Autodesk Fusion 360 part; units mm, degrees
(part 2 of 5)
  spline S0 degree 3 poles (45.4352, 19.4331, 2.5409) (44.7866, 20.9539, 2.7513) (44.0616, 22.4421, 2.9616) (43.2623, 23.8896, 3.172) (39.2446, 31.1652, 4.2293) (33.358, 37.3986, 5.2866) (26.324, 41.8256, 6.3439) (19.2902, 46.2525, 7.4011) (11.1241, 48.8637, 8.4584) (2.8268, 49.3391, 9.5157) (-5.4704, 49.8145, 10.5729) (-13.8811, 48.1531, 11.6302) (-21.3743, 44.5587, 12.6874) (-28.8674, 40.9643, 13.7447) (-35.4271, 35.4447, 14.8019) (-40.2493, 28.6763, 15.8591) (-45.0715, 21.908, 16.9163) (-48.146, 13.9055, 17.9735) (-49.096, 5.6496, 19.0307) (-50.046, -2.606, 20.0879) (-48.8696, -11.0975, 21.1451) (-45.711, -18.784, 22.2022) (-42.5525, -26.4703, 23.2594) (-37.4186, -33.3353, 24.3165) (-30.9385, -38.5376, 25.3737) (-24.4586, -43.7398, 26.4308) (-16.6463, -47.2683, 27.4879) (-8.4592, -48.6906, 28.545) (-0.2722, -50.113, 29.6021) (8.2721, -49.4263, 30.6592) (16.1268, -46.7147, 31.7163) (23.9813, -44.0032, 32.7734) (31.1295, -39.2726, 33.8305) (36.6953, -33.1027, 34.8876) (42.261, -26.933, 35.9446) (46.2326, -19.3372, 37.0017) (48.1234, -11.246, 38.0587) (50.0142, -3.155, 39.1157) (49.8203, 5.4141, 40.1728) (47.5655, 13.4113, 41.2298) (45.3107, 21.4083, 42.2868) (40.9999, 28.8164, 43.3438) (35.1612, 34.7279, 44.4008) (29.3227, 40.6393, 45.4577) (21.9688, 45.0415, 46.5147) (14.0006, 47.3954, 47.5717) (6.0326, 49.7491, 48.6286) (-2.5328, 50.0495, 49.6856) (-10.6461, 48.2597, 50.7425) (-18.7593, 46.4699, 51.7995) (-26.4031, 42.5939, 52.8564) (-32.6413, 37.1064, 53.9133) (-38.8792, 31.6191, 54.9702) (-43.6983, 24.5321, 56.0271) (-46.508, 16.7136, 57.084) (-49.3176, 8.8953, 58.1409) (-50.1121, 0.3622, 59.1978) (-48.7941, -7.8404, 60.2546) (-47.4761, -16.0429, 61.3115) (-44.0485, -23.8973, 62.3684) (-38.9312, -30.4418, 63.4252) (-33.8139, -36.986, 64.482) (-27.0179, -42.2064, 65.5389) (-19.3756, -45.4634, 66.5957) (-11.7334, -48.7204, 67.6525) (-3.2612, -50.0071, 68.7093) (5.0034, -49.1661, 69.7661) (13.2677, -48.3251, 70.8229) (21.3069, -45.3581, 71.8796) (28.1362, -40.6287, 72.9364) (34.9654, -35.8993, 73.9932) (40.5702, -29.4176, 75.0499) (44.2643, -21.9774, 76.1067) (47.9584, -14.5373, 77.1634) (49.7339, -6.1545, 78.2202) (49.3735, 2.1444, 79.2769) (49.013, 10.4431, 80.3336) (46.5175, 18.6401, 81.3903) (42.1925, 25.7318, 82.447) (37.8676, 32.8234, 83.5037) (31.7225, 38.7945, 84.5604) (24.5097, 42.914, 85.617) (17.2971, 47.0334, 86.6737) (9.0322, 49.2925, 87.7304) (0.7269, 49.4147, 88.787) (-7.5781, 49.5368, 89.8437) (-15.9057, 47.5219, 90.9003) (-23.2363, 43.6166, 91.9569) (-30.5667, 39.7114, 93.0135) (-36.8845, 33.9243, 94.0701) (-41.4161, 26.9637, 95.1268) (-45.9477, 20.0033, 96.1833) (-48.6835, 11.8843, 97.2399) (-49.2886, 3.6009, 98.2965) (-49.8938, -4.6824, 99.3531) (-48.3671, -13.1126, 100.4096) (-44.8954, -20.6576, 101.4662) (-41.4239, -28.2024, 102.5227) (-36.0148, -34.846, 103.5793) (-29.3305, -39.7751, 104.6358) (-22.6463, -44.7041, 105.6923) (-14.7012, -47.9081, 106.7488) (-6.4676, -48.995, 107.8054) (1.7658, -50.0818, 108.8619) (10.27, -49.0493, 109.9183) (18.0041, -46.0238, 110.9748) (25.738, -42.9983, 112.0313) (32.6854, -37.9864, 113.0878) (37.9957, -31.6016, 114.1442) (43.306, -25.2168, 115.2007) (46.9681, -17.4728, 116.2571) (48.5337, -9.3173, 117.3136) (50.0994, -1.1619, 118.37) (49.5653, 7.3875, 119.4264) (46.997, 15.2846, 120.4828) (44.4287, 23.1815, 121.5392) (39.8317, 30.4094, 122.5956) (33.7686, 36.0835, 123.652) (27.7056, 41.7575, 124.7084) (20.1894, 45.8659, 125.7648) (12.14, 47.9057, 126.8211) (4.0907, 49.9455, 127.8775) (-4.4747, 49.9126, 128.9338) (-12.508, 47.8109, 129.9902) (-20.5412, 45.7093, 131.0465) (-28.0252, 41.5436, 132.1029) (-34.0443, 35.8235, 133.1592) (-40.0632, 30.1035, 134.2155) (-44.6044, 22.8414, 135.2718) (-47.1122, 14.9259, 136.3281) (-49.6199, 7.0105, 137.3844) (-50.0889, -1.5416, 138.4407) (-48.462, -9.6838, 139.4969) (-46.835, -17.8258, 140.5532) (-43.1155, -25.5407, 141.6095) (-37.7587, -31.8844, 142.6657) (-32.402, -38.2281, 143.7219) (-25.4193, -43.1872, 144.7782) (-17.665, -46.155, 145.8344) (-9.911, -49.1227, 146.8906) (-1.4018, -50.093, 147.9468) (6.8213, -48.947, 149.0031) (15.0443, -47.801, 150.0592) (22.9638, -44.5413, 151.1154) (29.6109, -39.5668, 152.1716) (36.2579, -34.5923, 153.2278) (41.6184, -27.9136, 154.284) (45.0367, -20.3478, 155.3401) (48.4549, -12.782, 156.3963) (49.9237, -4.3452, 157.4524) (49.2634, 3.9305, 158.5085) (48.6032, 12.2061, 159.5647) (45.8153, 20.3031, 160.6208) (41.2409, 27.231, 161.6769) (36.6665, 34.1588, 162.733) (30.3154, 39.9028, 163.7891) (22.9644, 43.7604, 164.8452) (15.6136, 47.6179, 165.9013) (7.2785, 49.581, 166.9574) (-1.0213, 49.4094, 168.0134) (-9.3208, 49.2379, 169.0695) (-17.5675, 46.9322, 170.1255) (-24.7525, 42.7744, 171.1816) (-31.9374, 38.6166, 172.2376) (-38.0455, 32.6157, 173.2936) (-42.3297, 25.5055, 174.3497) (-46.6139, 18.3954, 175.4057) (-49.0651, 10.1912, 176.4617) (-49.3836, 1.8964, 177.5177) (-49.7021, -6.3984, 178.5737) (-47.8874, -14.7662, 179.6297) (-44.1613, -22.1837, 180.6857) (-40.4353, -29.6011, 181.7416) (-34.8059, -36.0525, 182.7976) (-27.9617, -40.749, 183.8535) (-21.1176, -45.4454, 184.9095) (-13.0731, -48.3769, 185.9654) (-4.8121, -49.1852, 187.0214) (3.4487, -49.9934, 188.0773) (11.9086, -48.6766, 189.1332) (19.5331, -45.396, 190.1891) (27.1574, -42.1154, 191.245) (33.9301, -36.8779, 192.3009) (39.023, -30.324, 193.3568) (44.1158, -23.7702, 194.4127) (47.5181, -15.9139, 195.4685) (48.814, -7.7157, 196.5244) (50.1098, 0.4823, 197.5803) (49.2964, 9.0047, 198.6361) (46.4733, 16.8097, 199.692) (43.6503, 24.6144, 200.7478) (38.8237, 31.685, 201.8036) (32.5835, 37.1571, 202.8595) (26.3435, 42.6291, 203.9153) (18.7032, 46.4909, 204.9711) (10.5968, 48.2705, 206.0269) (2.4906, 50.0501, 207.0827) (-6.0645, 49.7437, 208.1385) (-14.0227, 47.3888, 209.1942) (-21.9807, 45.034, 210.25) (-29.3248, 40.6358, 211.3058) (-35.1573, 34.7318, 212.3615) (-40.9897, 28.828, 213.4173) (-45.2981, 21.431, 214.473) (-47.5559, 13.4451, 215.5287) (-49.8137, 5.4594, 216.5845) (-50.0161, -3.0982, 217.6402) (-48.1384, -11.1818, 218.6959) (-46.2608, -19.2651, 219.7516) (-42.3071, -26.8572, 220.8073) (-36.7607, -33.0301, 221.863) (-31.2145, -39.2028, 222.9187) (-24.0873, -43.9432, 223.9744) (-16.2504, -46.6719, 225.03) (-8.4136, -49.4005, 226.0857) (0.1163, -50.1117, 227.1413) (8.2968, -48.7186, 228.197) (16.477, -47.3255, 229.2526) (24.2905, -43.8311, 230.3083) (30.7823, -38.6625, 231.3639) (37.2739, -33.4939, 232.4195) (42.4301, -26.6622, 233.4751) (45.6207, -19.0023, 234.5307) (48.8112, -11.3425, 235.5863) (50.0295, -2.8707, 236.6419) (49.1265, 5.3778, 237.6975) (48.2236, 13.6261, 238.7531) (45.2015, 21.6335, 239.8086) (40.4296, 28.4216, 240.8642) (35.6577, 35.2095, 241.9197) (29.1462, 40.7637, 242.9753) (21.6908, 44.4055, 244.0308) (14.2354, 48.0472, 245.0864) (5.852, 49.7688, 246.1419) (-2.4351, 49.36, 247.1974) (-10.7221, 48.9511, 248.2529) (-18.8952, 46.4128, 249.3084) (-25.9558, 42.0551, 250.3639) (-33.0162, 37.6976, 251.4194) (-38.9492, 31.5299, 252.4749) (-43.0298, 24.3059, 253.5304) (-47.1103, 17.082, 254.5858) (-49.3298, 8.817, 255.6413) (-49.4173, 0.5207, 256.6968) (-49.5047, -7.7753, 257.7522) (-47.4599, -16.0851, 258.8076) (-43.5326, -23.3933, 259.8631) (-39.6055, -30.7013, 260.9185) (-33.8043, -36.9923, 261.9739) (-26.8379, -41.4977, 263.0293) (-19.8716, -46.0031, 264.0847) (-11.7549, -48.7133, 265.1401) (-3.4792, -49.2974, 266.1955) (4.7962, -49.8814, 267.2509) (13.213, -48.3381, 268.3063) (20.7429, -44.8561, 269.3617) (28.2727, -41.3741, 270.417) (34.8997, -35.9607, 271.4724) (39.8143, -29.2773, 272.5277) (44.7288, -22.594, 273.5831) (47.9207, -14.6548, 274.6384) (49, -6.4296, 275.6937) (50.0792, 1.7954, 276.749) (49.0437, 10.2891, 277.8044) (46.0199, 18.0139, 278.8597) (42.9962, 25.7386, 279.915) (37.9907, 32.6781, 280.9703) (31.6148, 37.9848, 282.0256) (25.2389, 43.2914, 283.0808) (17.5063, 46.954, 284.1361) (9.3612, 48.5253, 285.1914) (1.2163, 50.0966, 286.2466) (-7.3237, 49.5733, 287.3019) (-15.2158, 47.0193, 288.3571) (-23.1077, 44.4654, 289.4124) (-30.3351, 39.8864, 290.4676) (-36.0152, 33.8414, 291.5228) (-41.6952, 27.7965, 292.578) (-45.816, 20.2986, 293.6333) (-47.8743, 12.2633, 294.6885) (-49.9325, 4.2281, 295.7437) (-49.924, -4.3274, 296.7988) (-47.8498, -12.3584, 297.854) (-45.7756, -20.3893, 298.9092) (-41.6402, -27.8788, 299.9644) (-35.9486, -33.9122, 301.0195) (-30.257, -39.9455, 302.0747) (-23.0213, -44.5101, 303.1298) (-15.1251, -47.0486, 304.185) (-7.229, -49.587, 305.2401) (1.311, -50.094, 306.2953) (9.452, -48.5077, 307.3504) (17.5928, -46.9214, 308.4055) (25.3175, -43.2452, 309.4606) (31.6828, -37.9281, 310.5157) (38.048, -32.611, 311.5708) (43.0403, -25.6642, 312.6259) (46.0504, -17.9359, 313.681) (49.0604, -10.2078, 314.736) (50.0817, -1.7145, 315.7911) (48.9898, 6.5069, 316.8462) (47.8978, 14.7282, 317.9012) (44.6949, 22.6602, 318.9563) (39.7721, 29.3346, 320.0113) (34.8494, 36.0088, 321.0664) (28.2172, 41.4114, 322.1214) (20.6853, 44.8827, 323.1764) (13.1536, 48.3539, 324.2314) (4.7381, 49.8865, 325.2864) (-3.5338, 49.2935, 326.3414) (-11.8056, 48.7005, 327.3964) (-19.9163, 45.9832, 328.4514) (-26.8757, 41.4733, 329.5064) (-33.8351, 36.9634, 330.5614) (-39.6286, 30.6706, 331.6163) (-43.5489, 23.3629, 332.6713) (-47.4692, 16.0554, 333.7263) (-49.5082, 7.7486, 334.7812) (-49.417, -0.5436, 335.8362) (-49.3258, -8.8356, 336.8911) (-47.1047, -17.0954, 337.946) (-43.0247, -24.3148, 339.0009) (-38.9448, -31.5341, 340.0558) (-33.0148, -37.6978, 341.1108) (-25.9585, -42.0534, 342.1657) (-18.9024, -46.409, 343.2206) (-10.7348, -48.9475, 344.2754) (-2.4529, -49.3591, 345.3303) (5.829, -49.7706, 346.3852) (14.2078, -48.0545, 347.4401) (21.6609, -44.4201, 348.4949) (29.1139, -40.7857, 349.5498) (35.6255, -35.2408, 350.6046) (40.401, -28.4622, 351.6595) (45.1764, -21.6836, 352.7143) (48.2057, -13.6857, 353.7692) (49.1192, -5.4444, 354.824) (50.0326, 2.7967, 355.8788) (48.8284, 11.2637, 356.9336) (45.6535, 18.9234, 357.9884) (42.4786, 26.5829, 359.0432) (37.3398, 33.4189, 360.098) (30.8642, 38.5971, 361.1528) (24.3887, 43.7753, 362.2076) (16.5901, 47.2848, 363.2623) (8.42, 48.6974, 364.3171) (0.2501, 50.11, 365.3719) (-8.274, 49.4229, 366.4266) (-16.1121, 46.7198, 367.4814) (-23.9501, 44.0167, 368.5361) (-31.0856, 39.3035, 369.5908) (-36.6479, 33.1552, 370.6456) (-42.2101, 27.0071, 371.7003) (-46.1875, 19.4369, 372.755) (-48.0946, 11.3684, 373.8097) (-50.0018, 3.3001, 374.8644) (-49.8349, -5.2495, 375.9191) (-47.6142, -13.2373, 376.9738) (-45.3936, -21.2249, 378.0285) (-41.1239, -28.6337, 379.0831) (-35.3263, -34.56, 380.1378) (-29.5287, -40.4861, 381.1925) (-22.2154, -44.9171, 382.2471) (-14.2786, -47.3123, 383.3018) (-6.3419, -49.7076, 384.3564) (2.2015, -50.0621, 385.4111) (10.3093, -48.3327, 386.4657) (18.417, -46.6034, 387.5203) (26.072, -42.7938, 388.5749) (32.3406, -37.3688, 389.6296) (38.609, -31.9438, 390.6842) (43.4777, -24.9149, 391.7388) (46.3527, -17.1395, 392.7933) (49.2277, -9.3642, 393.8479) (50.1031, -0.8589, 394.9025) (48.872, 7.339, 395.9571) (47.641, 15.5367, 397.0117) (44.3062, 23.4097, 398.0662) (39.2745, 29.9975, 399.1208) (34.2428, 36.5852, 400.1753) (27.5249, 41.874, 401.2299) (19.9401, 45.2187, 402.2844) (12.3555, 48.5633, 403.3389) (3.9201, 49.9568, 404.3935) (-4.3373, 49.2293, 405.448) (-12.5945, 48.5018, 406.5025) (-20.6562, 45.6549, 407.557) (-27.5391, 41.0358, 408.6115) (-34.4219, 36.4167, 409.666) (-40.1114, 30.0353, 410.7205) (-43.9137, 22.6698, 411.775) (-47.716, 15.3044, 412.8294) (-49.6231, 6.9705, 413.8839) (-49.4025, -1.3154, 414.9384) (-49.1819, -9.6012, 415.9928) (-46.834, -17.8217, 417.0473) (-42.6454, -24.9742, 418.1017) (-38.4567, -32.1266, 419.1561) (-32.4362, -38.196, 420.2106) (-25.3179, -42.4422, 421.265) (-18.1997, -46.6884, 422.3194) (-9.9988, -49.1025, 423.3738) (-1.7153, -49.3902, 424.4282) (6.568, -49.6779, 425.4826) (14.9165, -47.8386, 426.537) (22.312, -44.0966, 427.5914) (29.7074, -40.3547, 428.6458) (36.1343, -34.7181, 429.7002) (40.809, -27.874, 430.7546) (45.4837, -21.0301, 431.8089) (48.3963, -12.9933, 432.8633) (49.1918, -4.7435, 433.9176) (49.9873, 3.5061, 434.972) (48.6641, 11.9513, 436.0263) (45.3834, 19.5622, 437.0806) (42.1028, 27.173, 438.135) (36.8718, 33.9336, 439.1893) (30.3282, 39.0197, 440.2436) (23.7847, 44.1056, 441.2979) (15.9425, 47.5064, 442.3522) (7.7576, 48.8073, 443.4065) (-0.4271, 50.1082, 444.4608) (-8.9372, 49.3066, 445.5151) (-16.735, 46.5003, 446.5694) (-24.5327, 43.694, 447.6236) (-31.6018, 38.8888, 448.6779) (-37.0804, 32.6708, 449.7322) (-42.5589, 26.4528, 450.7864) (-46.4355, 18.835, 451.8407) (-48.2375, 10.7461, 452.8949) (-50.0395, 2.6574, 453.9492) (-49.7632, -5.8854, 455.0034) (-47.4423, -13.8408, 456.0576) (-45.1214, -21.7961, 457.1118) (-40.7609, -29.1472, 458.166) (-34.8923, -34.9981, 459.2203) (-29.0238, -40.8488, 460.2745) (-21.6597, -45.187, 461.3287) (-13.6976, -47.4838, 462.3829) (-5.7356, -49.7806, 463.437) (2.8075, -50.0312, 464.4912) (10.8904, -48.2051, 465.5454) (18.9732, -46.3791, 466.5995) (26.5788, -42.4803, 467.6537) (32.78, -36.9839, 468.7079) (38.9812, -31.4876, 469.762) (43.765, -24.4054, 470.8162) (46.5485, -16.6005, 471.8703) (49.3319, -8.7958, 472.9244) (50.109, -0.2849, 473.9785) (48.7853, 7.8949, 475.0327) (47.4616, 16.0746, 476.0868) (44.0398, 23.9058, 477.1409) (38.937, 30.4343, 478.195) (33.8343, 36.9626, 479.2491) (27.0614, 42.1743, 480.3032) (19.4437, 45.4343, 481.3573) (11.8261, 48.6943, 482.4113) (3.3799, 49.9957, 483.4654) (-4.8656, 49.1799, 484.5195) (-13.111, 48.3641, 485.5735) (-21.1384, 45.433, 486.6276) (-27.9694, 40.7437, 487.6816) (-34.8003, 36.0545, 488.7357) (-40.4205, 29.6171, 489.7897) (-44.1451, 22.2159, 490.8438) (-47.8696, 14.8149, 491.8978) (-49.6908, 6.4658, 492.9518) (-49.3867, -1.814, 494.0058) (-49.0826, -10.0937, 495.0598) (-46.6539, -18.2866, 496.1138) (-42.3965, -25.3944, 497.1678) (-38.1392, -32.502, 498.2218) (-32.0623, -38.5096, 499.2758) (-24.9063, -42.685, 500.3298) (-17.7504, -46.8604, 501.3838) (-9.5305, -49.195, 502.4377) (-1.2482, -49.4042, 503.4917) (7.034, -49.6135, 504.5457) (15.3612, -47.697, 505.5996) (22.7187, -43.8884, 506.6536) (30.0762, -40.0799, 507.7075) (36.4484, -34.3873, 508.7614) (41.0592, -27.5041, 509.8154) (45.6699, -20.6211, 510.8693) (48.5094, -12.5622, 511.9232) (49.2318, -4.3092, 512.9771) (49.9541, 3.9437, 514.031) (48.5579, 12.3733, 515.0849) (45.2132, 19.9525, 516.1388) (41.8685, 27.5317, 517.1927) (36.5825, 34.2445, 518.2466) (29.9991, 39.2733, 519.3005) (23.4158, 44.302, 520.3543) (15.549, 47.636, 521.4082) (7.3571, 48.8693, 522.4621) (-0.8346, 50.1025, 523.5159) (-9.3342, 49.2325, 524.5698) (-17.1061, 46.365, 525.6236) (-24.878, 43.4977, 526.6775) (-31.9058, 38.6391, 527.7313) (-37.3337, 32.3811, 528.7851) (-42.7614, 26.1232, 529.8389) (-46.5776, 18.4792, 530.8928) (-48.3176, 10.3802, 531.9466) (-50.0575, 2.2813, 533.0004) (-49.7174, -6.2555, 534.0542) (-47.3389, -14.1903, 535.108) (-44.9604, -22.125, 536.1618) (-40.5485, -29.441, 537.2156) (-34.6405, -35.2473, 538.2693) (-28.7326, -41.0535, 539.3231) (-21.3412, -45.3377, 540.3769) (-13.3665, -47.5781, 541.4306) (-5.392, -49.8184, 542.4844) (3.149, -50.0103, 543.5381) (11.2161, -48.1304, 544.5919) (19.2831, -46.2505, 545.6456) (26.8593, -42.3028, 546.6994) (33.0218, -36.7681, 547.7531) (39.1843, -31.2335, 548.8068) (43.9203, -24.1236, 549.8605) (46.653, -16.3044, 550.9143) (49.3857, -8.4852, 551.968) (50.1093, 0.0268, 553.0217) (48.7358, 8.195, 554.0754) (47.3623, 16.3631, 555.129) (43.8947, 24.1702, 556.1827) (38.7552, 30.6655, 557.2364) (33.6157, 37.1607, 558.2901) (26.8153, 42.3306, 559.3438) (19.182, 45.5454, 560.3974) (11.5489, 48.7602, 561.4511) (3.099, 50.0133, 562.5047) (-5.1386, 49.1521, 563.5584) (-13.3761, 48.2909, 564.612) (-21.3839, 45.3173, 565.6657) (-28.1871, 40.5934, 566.7193) (-34.9901, 35.8696, 567.7729) (-40.574, 29.4054, 568.8265) (-44.259, 21.9881, 569.8802) (-47.9439, 14.5709, 570.9338) (-49.7221, 6.2162, 571.9874) (-49.3771, -2.0588, 573.041) (-49.0321, -10.3336, 574.0946) (-46.5646, -18.5112, 575.1482) (-42.2752, -25.5958, 576.2017) (-37.9858, -32.6803, 577.2553) (-31.8835, -38.657, 578.3089) (-24.7113, -42.7982, 579.3625) (-17.5393, -46.9393, 580.416) (-9.3124, -49.2362, 581.4696) (-1.0325, -49.4092, 582.5231) (7.2473, -49.5822, 583.5767) (15.5628, -47.6311, 584.6302) (22.9015, -43.7933, 585.6838) (30.2402, -39.9556, 586.7373) (36.5866, -34.2395, 587.7908) (41.1682, -27.3407, 588.8443) (45.7497, -20.4421, 589.8979) (48.5568, -12.3755, 590.9514) (49.2477, -4.123, 592.0049) (49.9386, 4.1294, 593.0584) (48.5119, 12.5503, 594.1119) (45.1413, 20.1146, 595.1654) (41.7708, 27.6787, 596.2188) (36.4636, 34.3704, 597.2723) (29.8657, 39.3749, 598.3258) (23.2678, 44.3793, 599.3793) (15.3933, 47.686, 600.4327) (7.2007, 48.8926, 601.4862) (-0.9918, 50.0992, 602.5396) (-9.4852, 49.2031, 603.5931) (-17.2455, 46.3134, 604.6465) (-25.0058, 43.4237, 605.7) (-32.0166, 38.5466, 606.7534) (-37.4247, 32.2758, 607.8068) (-42.8328, 26.005, 608.8603) (-46.6267, 18.3537, 609.9137) (-48.3447, 10.2533, 610.9671) (-50.0626, 2.1529, 612.0205) (-49.7012, -6.3796, 613.0739) (-47.3042, -14.3056, 614.1273) (-44.9073, -22.2315, 615.1807) (-40.48, -29.5343, 616.2341) (-34.5612, -35.325, 617.2875) (-28.6425, -41.1158, 618.3408) (-21.2448, -45.3823, 619.3942) (-13.2686, -47.6055, 620.4476) (-5.2924, -49.8286, 621.5009) (3.2455, -50.0036, 622.5543) (11.3061, -48.1093, 623.6076) (19.3665, -46.2151, 624.661) (26.9327, -42.2555, 625.7143) (33.0837, -36.7125, 626.7677) (39.2345, -31.1696, 627.821) (43.9574, -24.055, 628.8743) (46.6773, -16.2346, 629.9277) (49.3973, -8.4143, 630.981) (50.1087, 0.0954, 632.0343) (48.725, 8.2588, 633.0876) (47.3414, 16.422, 634.1409) (43.8656, 24.2219, 635.1942) (38.7207, 30.709, 636.2475) (33.5759, 37.1961, 637.3008) (26.7728, 42.3569, 638.354) (19.1393, 45.5634, 639.4073) (11.506, 48.7699, 640.4606) (3.0583, 50.0153, 641.5139) (-5.1756, 49.1482, 642.5671) (-13.4094, 48.2812, 643.6204) (-21.4122, 45.3034, 644.6736) (-28.2102, 40.5774, 645.7269) (-35.008, 35.8514, 646.7801) (-40.5867, 29.3871, 647.8334) (-44.2675, 21.971, 648.8866) (-47.9482, 14.5551, 649.9398) (-49.7233, 6.203, 650.993) (-49.3767, -2.0688, 652.0463) (-49.0301, -10.3405, 653.0995) (-46.5627, -18.5147, 654.1527) (-42.2746, -25.5967, 655.2059) (-37.9867, -32.6786, 656.2591) (-31.8871, -38.6534, 657.3123) (-24.7182, -42.7942, 658.3655) (-17.5494, -46.935, 659.4186) (-9.3262, -49.2331, 660.4718) (-1.0493, -49.4089, 661.525) (7.2275, -49.5846, 662.5782) (15.5406, -47.6378, 663.6313) (22.8787, -43.8053, 664.6845) (30.2167, -39.9728, 665.7376) (36.5642, -34.2626, 666.7908) (41.149, -27.3696, 667.8439) (45.7337, -20.4766, 668.8971) (48.5461, -12.4153, 669.9502) (49.2441, -4.1664, 671.0033) (49.942, 4.0825, 672.0565) (48.524, 12.5016, 673.1096) (45.1626, 20.0668, 674.1627) (41.8013, 27.6318, 675.2158) (36.5037, 34.3271, 676.2689) (29.9143, 39.3379, 677.322) (23.325, 44.3487, 678.3751) (15.4578, 47.6647, 679.4282) (7.2698, 48.8824, 680.4813) (-0.9181, 50.1001, 681.5344) (-9.4097, 49.2171, 682.5875) (-17.1719, 46.3407, 683.6405) (-24.934, 43.4644, 684.6936) (-31.9504, 38.6009, 685.7467) (-37.3677, 32.3418, 686.7997) (-42.7849, 26.0828, 687.8528) (-46.5916, 18.4414, 688.9058) (-48.3247, 10.3471, 689.9589) (-50.0578, 2.2529, 691.0119) (-49.7137, -6.2772, 692.065) (-47.3344, -14.2055, 693.118) (-44.955, -22.1337, 694.171) (-40.5455, -29.4435, 695.224) (-34.642, -35.2458, 696.2771) (-28.7386, -41.0481, 697.3301) (-21.3538, -45.3306, 698.3831) (-13.3858, -47.5726, 699.4361) (-5.4179, -49.8146, 700.4891) (3.1165, -50.0114, 701.5421) (11.1792, -48.139, 702.5951) (19.2419, -46.2666, 703.6481) (26.816, -42.3291, 704.701) (32.9804, -36.8053, 705.754) (39.1447, -31.2816, 706.807) (43.8864, -24.1832, 707.86) (46.6288, -16.3736, 708.9129) (49.3711, -8.5641, 709.9659) (50.1083, -0.0597, 711.0188) (48.7508, 8.1052, 712.0718) (47.3269, 16.6698, 713.1763) (43.597, 24.8399, 714.2808) (38.0584, 31.5261, 715.3853) (32.5415, 38.1861, 716.4855) (25.2442, 43.3574, 717.5857) (17.1322, 46.3554, 718.6858) (9.0519, 49.3418, 719.7817) (0.1833, 50.1649, 720.8776) (-8.3086, 48.7166, 721.9735) (-16.7673, 47.2739, 723.0651) (-24.8317, 43.5816, 724.1567) (-31.4507, 38.1207, 725.2483) (-38.0438, 32.6812, 726.3357) (-43.187, 25.5004, 727.423) (-46.215, 17.5074, 728.5104) (-49.2311, 9.5456, 729.5935) (-50.1417, 0.7969, 730.6766) (-48.8297, -7.6154, 731.7597) (-47.5229, -15.9948, 732.8385) (-44.0143, -24.0209, 733.9174) (-38.751, -30.6707, 734.9963) (-33.5084, -37.2946, 736.0709) (-26.5371, -42.538, 737.1456) (-18.7189, -45.7377, 738.2202) (-10.9313, -48.9249, 739.2907) (-2.3212, -50.0775, 740.3611) (6.0305, -49.0507, 741.4316) (14.3495, -48.0279, 742.4979) (22.3937, -44.8454, 743.5641) (29.1608, -39.8997, 744.6304) (35.9014, -34.9733, 745.6925) (41.3602, -28.3085, 746.7546) (44.8623, -20.7295, 747.8167) (48.3506, -13.1802, 748.8747) (49.8902, -4.7401, 749.9326) (49.292, 3.5547, 750.9906) (48.6939, 11.8482, 752.0484) (45.96, 19.9789, 753.1062) (41.4257, 26.9489, 754.164) (36.8917, 33.9186, 755.2218) (30.5672, 39.7129, 756.2795) (23.2282, 43.621, 757.3372) (15.8895, 47.5288, 758.3949) (7.5521, 49.5422, 759.4526) (-0.7612, 49.4141, 760.5103) (-9.0741, 49.2861, 761.568) (-17.3451, 47.0171, 762.6256) (-24.5596, 42.8854, 763.6833) (-31.7739, 38.754, 764.7409) (-37.9163, 32.7689, 765.7985) (-42.2336, 25.6644, 766.856) (-46.5506, 18.5602, 767.9136) (-49.0335, 10.3518, 768.9711) (-49.3776, 2.0458, 770.0287) (-49.7218, -6.2597, 771.0862) (-47.9266, -14.645, 772.1436) (-44.2124, -22.0817, 773.2011) (-40.4984, -29.518, 774.2586) (-34.8733, -35.99, 775.316) (-28.0271, -40.704, 776.3734) (-21.1812, -45.4179, 777.4308) (-13.1288, -48.3638, 778.4882) (-4.8572, -49.1807, 779.5456) (3.414, -49.9976, 780.6029) (11.8867, -48.6839, 781.6603) (19.5222, -45.4007, 782.7176) (27.1573, -42.1176, 783.7749) (33.939, -36.8722, 784.8322) (39.0358, -30.3075, 785.8895) (44.1324, -23.7431, 786.9467) (47.5335, -15.8735, 788.0039) (48.8222, -7.6634, 789.0612) (50.1109, 0.5463, 790.1183) (49.2846, 9.0791, 791.1755) (46.4446, 16.889, 792.2327) (43.6047, 24.6985, 793.2898) (38.7575, 31.7687, 794.347) (32.4969, 37.2329, 795.4041) (26.2365, 42.6969, 796.4612) (18.5763, 46.5436, 797.5183) (10.4549, 48.3015, 798.5754) (2.3339, 50.0593, 799.6324) (-6.2309, 49.7248, 800.6894) (-14.1901, 47.339, 801.7465) (-22.1489, 44.9533, 802.8034) (-29.4851, 40.5216, 803.8604) (-35.3, 34.5868, 804.9174) (-41.1146, 28.6523, 805.9743) (-45.3955, 21.2275, 807.0313) (-47.6184, 13.2221, 808.0882) (-49.8411, 5.2171, 809.1451) (-50.0013, -3.3515, 810.202) (-48.0791, -11.434, 811.2589) (-46.157, -19.5161, 812.3157) (-42.157, -27.0949, 813.3725) (-36.569, -33.2422, 814.4294) (-30.9812, -39.3892, 815.4862) (-23.8175, -44.0916, 816.543) (-15.9552, -46.7736, 817.5997) (-8.0933, -49.4554, 818.6565) (0.4504, -50.1112, 819.7132) (8.6296, -48.6607, 820.77) (16.8083, -47.2103, 821.8267) (24.6051, -43.6568, 822.8833) (31.0653, -38.4355, 823.94) (37.5251, -33.2143, 824.9967) (42.6346, -26.3366, 826.0533) (45.7682, -18.6443, 827.11) (48.9016, -10.9525, 828.1666) (50.0525, -2.4625, 829.2232) (49.0801, 5.786, 830.2798) (48.1078, 14.0341, 831.3363) (45.0143, 22.0233, 832.3928) (40.1785, 28.7755, 833.4494) (35.3428, 35.5273, 834.5059) (28.7753, 41.0279, 835.5624) (21.2797, 44.6039, 836.6189) (13.7845, 48.1798, 837.6754) (5.3773, 49.8235, 838.7318) (-2.9127, 49.3341, 839.7883) (-11.2024, 48.8447, 840.8447) (-19.3574, 46.2232, 841.9011) (-26.3796, 41.7906, 842.9575) (-33.4014, 37.3582, 844.0138) (-39.2756, 31.1242, 845.0702) (-43.2833, 23.8515, 846.1266) (-47.2907, 16.5792, 847.1829) (-49.4233, 8.2838, 848.2392) (-49.42, -0.0196, 849.2955) (-49.4167, -8.3227, 850.3518) (-47.2777, -16.616, 851.408) (-43.2648, -23.8849, 852.4643) (-39.2521, -31.1535, 853.5205) (-33.3741, -37.3823, 854.5767) (-26.3501, -41.8092, 855.633) (-19.3263, -46.2359, 856.6891) (-11.1715, -48.8514, 857.7453) (-2.8834, -49.3358, 858.8015) (5.4044, -49.8202, 859.8576) (13.808, -48.1726, 860.9137) (21.2994, -44.5945, 861.9699) (28.7904, -41.0167, 863.026) (35.3533, -35.5161, 864.082) (40.1854, -28.7657, 865.1381) (45.0173, -22.0157, 866.1942) (48.1082, -14.0302, 867.2502) (49.0801, -5.786, 868.3062) (50.052, 2.4578, 869.3622) (48.9029, 10.9427, 870.4182) (45.7735, 18.6311, 871.4742) (42.6443, 26.3192, 872.5302) (37.5414, 33.1945, 873.5861) (31.0891, 38.4162, 874.6421) (24.637, 43.6377, 875.698) (16.8492, 47.1946, 876.7539) (8.678, 48.6521, 877.8098) (0.5071, 50.1095, 878.8656) (-8.0298, 49.4646, 879.9215) (-15.889, 46.7961, 880.9774) (-23.7478, 44.1277, 882.0332) (-30.9123, 39.4417, 883.089) (-36.5065, 33.3109, 884.1448) (-42.1004, 27.1803, 885.2006) (-46.1123, 19.6181, 886.2564) (-48.0517, 11.5487, 887.3121) (-49.991, 3.4797, 888.3678) (-49.8539, -5.0793, 889.4236) (-47.6571, -13.0821, 890.4793) (-45.4604, -21.0845, 891.535) (-41.2088, -28.5138, 892.5907) (-35.4221, -34.4617, 893.6464) (-29.6356, -40.4095, 894.702) (-22.3264, -44.8634, 895.7576) (-14.3877, -47.2793, 896.8133) (-6.4494, -49.695, 897.8689) (2.1015, -50.0677, 898.9245) (10.2199, -48.3517, 899.9801) (18.338, -46.6358, 901.0356) (26.0065, -42.8351, 902.0912) (32.2882, -37.4141, 903.1467) (38.5696, -31.9932, 904.2023) (43.4511, -24.9636, 905.2578) (46.3361, -17.1843, 906.3133) (49.2211, -9.4052, 907.3687) (50.1036, -0.8929, 908.4242) (48.876, 7.3125, 909.4797) (47.6484, 15.5176, 910.5351) (44.3134, 23.3986, 911.5905) (39.2784, 29.9925, 912.646) (34.2435, 36.5861, 913.7014) (27.5195, 41.8788, 914.7567) (19.9278, 45.2241, 915.8121) (12.3363, 48.5692, 916.8675) (3.8933, 49.96, 917.9228) (-4.37, 49.2264, 918.9782) (-12.633, 48.4929, 920.0335) (-20.6987, 45.6368, 921.0888) (-27.582, 41.007, 922.1441) (-34.465, 36.3774, 923.1993) (-40.151, 29.984, 924.2546) (-43.9457, 22.6077, 925.3098) (-47.7403, 15.2317, 926.3651) (-49.6356, 6.8885, 927.4203) (-49.4001, -1.4029, 928.4755) (-49.1646, -9.6941, 929.5307) (-46.7991, -17.9159, 930.5859) (-42.5923, -25.0645, 931.641) (-38.3858, -32.2128, 932.6962) (-32.347, -38.2727, 933.7513) (-25.2135, -42.5043, 934.8064) (-18.0803, -46.7357, 935.8615) (-9.8675, -49.13, 936.9166) (-1.5779, -49.3948, 937.9717) (6.7114, -49.6596, 939.0268) (15.06, -47.7945, 940.0818) (22.4485, -44.0273, 941.1369) (29.8367, -40.2602, 942.1919) (36.2494, -34.599, 943.2469) (40.9036, -27.735, 944.302) (45.5577, -20.8711, 945.3569) (48.4436, -12.819, 946.4119) (49.209, -4.5615, 947.4669) (49.9744, 3.6957, 948.5218) (48.618, 12.1407, 949.5768) (45.3051, 19.7428, 950.6317) (41.9925, 27.3447, 951.6866) (36.7306, 34.0875, 952.7415) (30.1618, 39.1485, 953.7964) (23.5933, 44.2092, 954.8512) (15.7318, 47.5774, 955.9061) (7.5368, 48.8419, 956.961) (-0.6579, 50.1064, 958.0158) (-9.1687, 49.2648, 959.0706) (-16.9569, 46.4198, 960.1254) (-24.7449, 43.5749, 961.1802) (-31.794, 38.7327, 962.235) (-37.244, 32.4842, 963.2897) (-42.6938, 26.2359, 964.3445) (-46.533, 18.5945, 965.3992) (-48.2933, 10.4925, 966.454) (-50.0535, 2.3907, 967.5087) (-49.7312, -6.1545, 968.5634) (-47.3657, -14.1006, 969.6181) (-45.0003, -22.0464, 970.6727) (-40.5968, -29.3764, 971.7274) (-34.6924, -35.1962, 972.7821) (-28.7883, -41.0158, 973.8367) (-21.3959, -45.3131, 974.8913) (-13.4172, -47.5638, 975.9459) (-5.4387, -49.8144, 977.0005) (3.1093, -50.0139, 978.0551) (11.1841, -48.1379, 979.1097) (19.2586, -46.2619, 980.1643) (26.8428, -42.3145, 981.2188) (33.0117, -36.7772, 982.2734) (39.1804, -31.2402, 983.3279) (43.9208, -24.125, 984.3824) (46.6547, -16.2996, 985.4369) (49.3885, -8.4744, 986.4914) (50.1103, 0.0444, 987.5458) (48.7319, 8.218, 988.6003) (47.3536, 16.3912, 989.6548) (43.8783, 24.202, 990.7092) (38.7297, 30.6977, 991.7636) (33.5813, 37.1932, 992.818) (26.7706, 42.36, 993.8724) (19.1283, 45.568, 994.9268) (11.4862, 48.776, 995.9812) (3.0286, 50.0186, 997.0356) (-5.2133, 49.1443, 998.0899) (-13.4548, 48.27, 999.1443) (-21.4633, 45.2808, 1000.1986) (-28.2621, 40.5412, 1001.2529) (-35.0607, 35.8018, 1002.3072) (-40.6354, 29.3221, 1003.3615) (-44.3066, 21.892, 1004.4158) (-47.9777, 14.4623, 1005.4701) (-49.7376, 6.098, 1006.5243) (-49.3718, -2.1812, 1007.5786) (-49.0061, -10.4601, 1008.6328) (-46.5156, -18.6363, 1009.687) (-42.2038, -25.7133, 1010.7412) (-37.8923, -32.7899, 1011.7954) (-31.7688, -38.7524, 1012.8496) (-24.5797, -42.8739, 1013.9038) (-17.3909, -46.9953, 1014.9579) (-9.1518, -49.2671, 1016.0121) (-0.8667, -49.4124, 1017.0662) (7.4181, -49.5577, 1018.1204) (15.7316, -47.5764, 1019.1745) (23.0603, -43.7099, 1020.2286) (30.3888, -39.8436, 1021.2827) (36.7172, -34.1004, 1022.3367) (41.2743, -27.1803, 1023.3908) (45.8312, -20.2604, 1024.4449) (48.6074, -12.1782, 1025.4989) (49.2644, -3.9188, 1026.553) (49.9214, 4.3404, 1027.607) (48.458, 12.7596, 1028.661) (45.0525, 20.3127, 1029.715) (41.6472, 27.8655, 1030.769) (36.3072, 34.5365, 1031.8229) (29.683, 39.5127, 1032.8769) (23.0591, 44.4888, 1033.9309) (15.1652, 47.7597, 1034.9848) (6.9631, 48.927, 1036.0387) (-1.2387, 50.0943, 1037.0926) (-9.7315, 49.1555, 1038.1466) (-17.4804, 46.2252, 1039.2005) (-25.2291, 43.295, 1040.2543) (-32.2177, 38.3794, 1041.3082) (-37.5949, 32.0775, 1042.3621) (-42.9718, 25.7757, 1043.4159) (-46.726, 18.1008, 1044.4698) (-48.4002, 9.9877, 1045.5236) (-50.0744, 1.875, 1046.5774) (-49.665, -6.6588, 1047.6312) (-47.2221, -14.5741, 1048.685) (-44.7793, -22.4892, 1049.7388) (-40.3082, -29.7691, 1050.7926) (-34.3534, -35.5272, 1051.8463) (-28.3987, -41.2851, 1052.9001) (-20.973, -45.5091, 1053.9538) (-12.9807, -47.6848, 1055.0076) (-4.9886, -49.8604, 1056.0613) (3.5533, -49.9832, 1057.115) (11.6047, -48.0382, 1058.1687) (19.6557, -46.0933, 1059.2224) (27.1994, -42.0848, 1060.276) (33.3169, -36.501, 1061.3297) (39.4342, -30.9174, 1062.3834) (44.1125, -23.7702, 1063.437) (46.7822, -15.9298, 1064.4907) (49.4519, -8.0897, 1065.5443) (50.1074, 0.427, 1066.5979) (48.6689, 8.5833, 1067.6515) (47.2305, 16.7394, 1068.7051) (43.7013, 24.5178, 1069.7586) (38.511, 30.9716, 1070.8122) (33.3208, 37.4252, 1071.8658) (26.4807, 42.5405, 1072.9193) (18.8232, 45.6949, 1073.9729) (11.166, 48.8491, 1075.0264) (2.7078, 50.0359, 1076.0799) (-5.5218, 49.1105, 1077.1334) (-13.7511, 48.1853, 1078.1869) (-21.7345, 45.1501, 1079.2404) (-28.4999, 40.3744, 1080.2939) (-35.2651, 35.5989, 1081.3473) (-40.7983, 29.0931, 1082.4008) (-44.4259, 21.649, 1083.4542) (-48.0533, 14.2051, 1084.5077) (-49.7676, 5.8386, 1085.5611) (-49.3601, -2.432, 1086.6145) (-48.9526, -10.7024, 1087.6679) (-46.4243, -18.8597, 1088.7213) (-42.0829, -25.9108, 1089.7747) (-37.7416, -32.9616, 1090.8281) (-31.5965, -38.8917, 1091.8814) (-24.3954, -42.9791, 1092.9348) (-17.1946, -47.0664, 1093.9881) (-8.953, -49.3025, 1095.0414) (-0.6738, -49.4154, 1096.0948) (7.6052, -49.5283, 1097.1481) (15.9044, -47.5178, 1098.2014) (23.2138, -43.6286, 1099.2547) (30.5231, -39.7395, 1100.308) (36.8273, -33.98, 1101.3612) (41.3592, -27.0509, 1102.4145) (45.891, -20.1221, 1103.4677) (48.6412, -12.0383, 1104.521) (49.275, -3.7833, 1105.5742) (49.9088, 4.4714, 1106.6274) (48.425, 12.88, 1107.6807) (45.0043, 20.4193, 1108.7339) (41.5837, 27.9584, 1109.7871) (36.2333, 34.6124, 1110.8402) (29.6043, 39.5717, 1111.8934) (22.9755, 44.5309, 1112.9466) (15.0819, 47.785, 1113.9997) (6.884, 48.9382, 1115.0529) (-1.3136, 50.0913, 1116.106) (-9.7983, 49.1412, 1117.1591) (-17.5379, 46.2034, 1118.2123) (-25.2772, 43.2657, 1119.2654) (-32.2552, 38.3467, 1120.3185) (-37.6228, 32.0446, 1121.3716) (-42.9904, 25.7428, 1122.4246) (-46.7364, 18.0712, 1123.4777) (-48.4053, 9.9633, 1124.5308) (-50.0741, 1.8556, 1125.5838) (-49.6623, -6.6715, 1126.6369) (-47.2201, -14.5807, 1127.6899) (-44.7779, -22.4897, 1128.7429) (-40.3105, -29.7643, 1129.7959) (-34.3613, -35.5195, 1130.8489) (-28.4122, -41.2746, 1131.9019) (-20.9938, -45.4984, 1132.9549) (-13.0085, -47.6772, 1134.0079) (-5.0233, -49.8559, 1135.0609) (3.512, -49.9851, 1136.1138) (11.5594, -48.0491, 1137.1668) (19.9816, -46.0229, 1138.2688) (27.8484, -41.7353, 1139.3707) (34.1157, -35.7555, 1140.4727) (40.334, -29.8223, 1141.5661) (44.9628, -22.2385, 1142.6595) (47.3968, -13.9956, 1143.7529) (49.8118, -5.8171, 1144.8377) (50.0611, 2.9904, 1145.9225) (48.1126, 11.2924, 1147.0074) (46.1792, 19.5295, 1148.0837) (42.0875, 27.2501, 1149.1601) (36.3565, 33.4745, 1150.2364) (30.6702, 39.6503, 1151.3044) (23.3835, 44.3399, 1152.3723) (15.407, 46.957, 1153.4403) (7.4928, 49.5537, 1154.4999) (-1.083, 50.1053, 1155.5595) (-9.2646, 48.5438, 1156.6191) (-17.432, 46.9851, 1157.6769) (-25.1892, 43.3241, 1158.7346) (-31.5843, 38.0101, 1159.7924) (-37.9789, 32.6966, 1160.8501) (-42.9979, 25.7417, 1161.9077) (-46.0259, 17.9987, 1162.9654) (-49.0536, 10.2564, 1164.023) (-50.084, 1.7427, 1165.0805) (-48.9909, -6.4984, 1166.1381) (-47.8979, -14.7386, 1167.1955) (-44.684, -22.6886, 1168.253) (-39.7435, -29.3734, 1169.3105) (-34.8034, -36.0575, 1170.3678) (-28.1474, -41.4625, 1171.4252) (-20.5917, -44.9257, 1172.4825) (-13.0367, -48.3885, 1173.5398) (-4.5982, -49.9025, 1174.597) (3.6894, -49.2821, 1175.6543) (11.9762, -48.6617, 1176.7114) (20.0945, -45.9086, 1177.7686) (27.0493, -41.3603, 1178.8257) (34.0034, -36.8124, 1179.8828) (39.7794, -30.4792, 1180.9398) (43.6695, -23.1368, 1181.9969) (47.5592, -15.7952, 1183.0539) (49.5551, -7.4602, 1184.1108) (49.4127, 0.8471, 1185.1678) (49.2703, 9.1535, 1186.2246) (46.9903, 17.4145, 1187.2815) (42.8519, 24.618, 1188.3383) (38.7139, 31.8209, 1189.3951) (32.7268, 37.9513, 1190.4518) (25.6236, 42.2583, 1191.5086) (18.5212, 46.5649, 1192.5653) (10.3181, 49.0394, 1193.6219) (2.0189, 49.3787, 1194.6786) (-6.2796, 49.718, 1195.7352) (-14.6565, 47.9218, 1196.7917) (-22.0863, 44.2101, 1197.8483) (-29.5155, 40.4986, 1198.9048) (-35.9819, 34.8799, 1199.9612) (-40.6941, 28.0415, 1201.0177) (-45.4058, 21.2038, 1202.0741) (-48.3536, 13.1613, 1203.1305) (-49.1767, 4.8983, 1204.1868) (-49.9996, -3.364, 1205.2431) (-48.6965, -11.8293, 1206.2994) (-45.4267, -19.4615, 1207.3557) (-42.1572, -27.0931, 1208.4119) (-36.9284, -33.8757, 1209.4681) (-30.3799, -38.9795, 1210.5243) (-23.832, -44.0828, 1211.5804) (-15.9786, -47.4967, 1212.6365) (-7.7804, -48.8037, 1213.6926) (0.4171, -50.1106, 1214.7486) (8.942, -49.3081, 1215.8046) (16.7516, -46.4943, 1216.8606) (24.5605, -43.6808, 1217.9165) (31.6378, -38.8624, 1218.9725) (37.1178, -32.6282, 1220.0284) (42.5975, -26.3946, 1221.0842) (46.4686, -18.7588, 1222.1401) (48.2579, -10.6544, 1223.1959) (50.047, -2.5506, 1224.2516) (49.7509, 6.0046, 1225.3074) (47.4058, 13.9653, 1226.3631) (45.0608, 21.9253, 1227.4188) (40.6721, 29.2741, 1228.4744) (34.7761, 35.1135, 1229.5301) (28.8806, 40.9524, 1230.5857) (21.4905, 45.2697, 1231.6412) (13.509, 47.5378, 1232.6968) (5.528, 49.8058, 1233.7523) (-3.0273, 50.0201, 1234.8078) (-11.1118, 48.1546, 1235.8633) (-19.1956, 46.2892, 1236.9187) (-26.7915, 42.3483, 1237.9741) (-32.9714, 36.8134, 1239.0295) (-39.1508, 31.2788, 1240.0848) (-43.9015, 24.1622, 1241.1401) (-46.6431, 16.3327, 1242.1954) (-49.3845, 8.5039, 1243.2507) (-50.1113, -0.0211, 1244.3059) (-48.7348, -8.201, 1245.3611) (-47.3584, -16.3803, 1246.4163) (-43.8819, -24.1973, 1247.4714) (-38.7299, -30.6974, 1248.5266) (-33.5783, -37.1971, 1249.5817) (-26.7622, -42.3663, 1250.6367) (-19.114, -45.574, 1251.6918) (-11.4664, -48.7815, 1252.7468) (-3.0029, -50.0209, 1253.8018) (5.2434, -49.1411, 1254.8568) (13.4889, -48.2613, 1255.9117) (21.4998, -45.2643, 1256.9666) (28.2982, -40.516, 1258.0215) (35.096, -35.7681, 1259.0764) (40.6672, -29.2792, 1260.1312) (44.3317, -21.8411, 1261.186) (47.996, -14.4036, 1262.2408) (49.7462, -6.0329, 1263.2955) (49.3688, 2.2497, 1264.3503) (48.9914, 10.5317, 1265.405) (46.4874, 18.708, 1266.4597) (42.1625, 25.781, 1267.5143) (37.8378, 32.8536, 1268.5689) (31.7016, 38.8081, 1269.6235) (24.5023, 42.9182, 1270.6781) (17.3034, 47.0281, 1271.7327) (9.0569, 49.2851, 1272.7872) (0.7686, 49.414, 1273.8417) (-7.5192, 49.5429, 1274.8962) (-15.8313, 47.5438, 1275.9506) (-23.1541, 43.6603, 1277.0051) (-30.4764, 39.7772, 1278.0595) (-36.7939, 34.0182, 1279.1138) (-41.3365, 27.0857, 1280.1682) (-45.8787, 20.1536, 1281.2225) (-48.6365, 12.0628, 1282.2768) (-49.2737, 3.7997, 1283.3311) (-49.9109, -4.4628, 1284.3854) (-48.4264, -12.8802, 1285.4396) (-45.0012, -20.4263, 1286.4938) (-41.5762, -27.9718, 1287.548) (-36.218, -34.6303, 1288.6022) (-29.5797, -39.5901, 1289.6563) (-22.9419, -44.5496, 1290.7104) (-15.0381, -47.8001, 1291.7645) (-6.8317, -48.9455, 1292.8186) (1.3741, -50.0909, 1293.8726) (9.8653, -49.129, 1294.9267) (17.607, -46.1771, 1295.9807) (25.3483, -43.2255, 1297.0346) (32.3239, -38.2903, 1298.0886) (37.6838, -31.9729, 1299.1426) (43.0435, -25.6559, 1300.1964) (46.7765, -17.9702, 1301.2503) (48.428, -9.8521, 1302.3042) (50.0794, -1.7346, 1303.358) (49.6462, 6.7981, 1304.4119) (47.181, 14.7066, 1305.4657) (44.7161, 22.6147, 1306.5194) (40.2246, 29.8819, 1307.5732) (34.2538, 35.6232, 1308.6269) (28.2834, 41.3641, 1309.6806) (20.8463, 45.5672, 1310.7343) (12.8484, 47.7206, 1311.788) (4.8509, 49.8738, 1312.8416) (-3.6905, 49.9731, 1313.8953) (-11.7359, 48.0063, 1314.9489) (-19.7807, 46.0396, 1316.0024) (-27.3126, 42.0112, 1317.056) (-33.4145, 36.4117, 1318.1096) (-39.5159, 30.8124, 1319.1631) (-44.1747, 23.654, 1320.2166) (-46.8236, 15.8078, 1321.2701) (-49.4724, 7.962, 1322.3235) (-50.1059, -0.5549, 1323.3769) (-48.6471, -8.7061, 1324.4304) (-47.1884, -16.8569, 1325.4837) (-43.6407, -24.625, 1326.5371) (-38.4357, -31.0649, 1327.5905) (-33.2311, -37.5045, 1328.6438) (-26.3804, -42.6024, 1329.6971) (-18.7174, -45.7383, 1330.7504) (-11.0549, -48.8741, 1331.8037) (-2.5962, -50.0414, 1332.8569) (5.6293, -49.0983, 1333.9102) (13.8543, -48.1553, 1334.9634) (21.8289, -45.1041, 1336.0166) (28.5826, -40.3159, 1337.0698) (35.336, -35.5279, 1338.1229) (40.8546, -29.0133, 1339.1761) (44.4669, -21.5645, 1340.2292) (48.079, -14.1162, 1341.2823) (49.7776, -5.7495, 1342.3354) (49.3558, 2.5177, 1343.3884) (48.9341, 10.7846, 1344.4415) (46.3933, 18.9346, 1345.4945) (42.0424, 25.9764, 1346.5475) (37.6917, 33.0179, 1347.6005) (31.5403, 38.9365, 1348.6534) (24.3364, 43.0125, 1349.7064) (16.8312, 47.2589, 1350.8034) (8.1992, 49.4921, 1351.9004) (-0.4236, 49.4182, 1352.9974) (-8.9118, 49.3454, 1354.0772) (-17.3709, 47.0387, 1355.1571) (-24.721, 42.7926, 1356.2369) (-31.9563, 38.6129, 1357.2999) (-38.1014, 32.5643, 1358.3629) (-42.3954, 25.3962, 1359.4259) (-46.668, 18.2637, 1360.4836) (-49.0989, 10.0382, 1361.5413) (-49.3897, 1.729, 1362.599) (-49.6806, -6.5787, 1363.6565) (-47.8316, -14.9523, 1364.714) (-44.0697, -22.3651, 1365.7715) (-40.3085, -29.7764, 1366.8288) (-34.6431, -36.2115, 1367.8861) (-27.7679, -40.8813, 1368.9434) (-20.8941, -45.5502, 1370.0005) (-12.8257, -48.4447, 1371.0576) (-4.5515, -49.21, 1372.1147) (3.7212, -49.9751, 1373.1716) (12.182, -48.6103, 1374.2285) (19.7944, -45.2826, 1375.2853) (27.4055, -41.9556, 1376.342) (34.1523, -36.6736, 1377.3987) (39.2087, -30.0835, 1378.4555) (44.2642, -23.4945, 1379.512) (47.6191, -15.6119, 1380.5685) (48.8627, -7.4006, 1381.625) (50.1062, 0.8092, 1382.6813) (49.2365, 9.3302, 1383.7376) (46.3601, 17.1195, 1384.7939) (43.4842, 24.9075, 1385.8501) (38.6084, 31.9476, 1386.9062) (32.3292, 37.3786, 1387.9624) (26.0511, 42.8086, 1389.0183) (18.3833, 46.6185, 1390.0743) (10.2637, 48.3424, 1391.1302) (2.1455, 50.0661, 1392.186) (-6.4073, 49.7007, 1393.2418) (-14.349, 47.291, 1394.2976) (-22.2894, 44.8818, 1395.3532) (-29.6021, 40.434, 1396.4088) (-35.3933, 34.4913, 1397.4644) (-41.1836, 28.5496, 1398.5198) (-45.4407, 21.126, 1399.5753) (-47.6446, 13.1275, 1400.6307) (-49.848, 5.1303, 1401.686) (-49.9942, -3.4246, 1402.7412) (-48.0652, -11.4924, 1403.7965) (-46.1365, -19.5589, 1404.8516) (-42.1374, -27.1214, 1405.9067) (-36.5561, -33.2564, 1406.9618) (-30.9757, -39.3905, 1408.0168) (-23.8255, -44.0846, 1409.0717) (-15.9782, -46.7657, 1410.1266) (-8.1321, -49.4465, 1411.1814) (0.3942, -50.1092, 1412.2362) (8.5603, -48.673, 1413.291) (16.7251, -47.237, 1414.3456) (24.5126, -43.7058, 1415.4003) (30.9727, -38.5101, 1416.4549) (37.4319, -33.3152, 1417.5094) (42.5503, -26.4673, 1418.5639) (45.7038, -18.8015, 1419.6184) (48.8569, -11.1369, 1420.6727) (50.0389, -2.6709, 1421.727) (49.1058, 5.5643, 1422.7814) (48.1727, 13.7983, 1423.8356) (45.1271, 21.7842, 1424.8897) (40.3401, 28.5484, 1425.9439) (35.5538, 35.3117, 1426.998) (29.0366, 40.8395, 1428.052) (21.5829, 44.458, 1429.1061) (14.1302, 48.0761, 1430.16) (5.7568, 49.7778, 1431.2139) (-2.517, 49.3559, 1432.2678) (-10.7897, 48.934, 1433.3216) (-18.9455, 46.3899, 1434.3754) (-25.9909, 42.0334, 1435.4292) (-33.0354, 37.6775, 1436.4828) (-38.955, 31.5189, 1437.5365) (-43.0288, 24.3076, 1438.5901) (-47.1021, 17.0971, 1439.6436) (-49.3215, 8.8493, 1440.6972) (-49.4167, 0.5684, 1441.7507) (-49.512, -7.7116, 1442.8041) (-47.4834, -16.0072, 1443.8575) (-43.5779, -23.3089, 1444.9109) (-39.6729, -30.6097, 1445.9642) (-33.8996, -36.9013, 1447.0174) (-26.9606, -41.4181, 1448.0707) (-20.0224, -45.9345, 1449.1239) (-11.9334, -48.6669, 1450.177) (-3.6777, -49.283, 1451.2302) (4.5771, -49.899, 1452.2833) (12.9811, -48.3978, 1453.3363) (20.5122, -44.9621, 1454.3893) (28.4043, -41.3616, 1455.4929) (35.3172, -35.641, 1456.5964) (40.3306, -28.5619, 1457.7) (45.1873, -21.7039, 1458.769) (48.2525, -13.5887, 1459.8381) (49.1422, -5.2323, 1460.9071) (50.0224, 3.0342, 1461.9647) (48.7726, 11.5186, 1463.0223) (45.5462, 19.1803, 1464.0798) (42.3209, 26.839, 1465.137) (37.1275, 33.6592, 1466.1942) (30.6023, 38.8051, 1467.2513) (24.0796, 43.949, 1468.3081) (16.2401, 47.4089, 1469.3649) (8.0439, 48.761, 1470.4216) (-0.1494, 50.1126, 1471.478) (-8.6816, 49.3551, 1472.5344) (-16.5086, 46.5811, 1473.5908) (-24.3328, 43.8082, 1474.6468) (-31.4357, 39.0261, 1475.7028) (-36.9485, 32.8199, 1476.7589) (-42.4594, 26.6157, 1477.8145) (-46.3696, 19.0014, 1478.8702) (-48.2012, 10.9078, 1479.9259) (-50.0322, 2.8167, 1480.9812) (-49.782, -5.7363, 1482.0365) (-47.4812, -13.7065, 1483.0918) (-45.1812, -21.6742, 1484.1468) (-40.8367, -29.0427, 1485.2018) (-34.9781, -34.9123, 1486.2568) (-29.1213, -40.7802, 1487.3115) (-21.7637, -45.1377, 1488.3662) (-13.803, -47.4533, 1489.4209) (-5.8446, -49.7682, 1490.4753) (2.6998, -50.0374, 1491.5297) (10.7882, -48.2281, 1492.584) (18.8743, -46.4193, 1493.6381) (26.4877, -42.537, 1494.6922) (32.7004, -37.0543, 1495.7463) (38.9115, -31.573, 1496.8002) (43.7096, -24.5037, 1497.854) (46.5101, -16.7076, 1498.9078) (49.31, -8.9134, 1499.9614) (50.1075, -0.4092, 1501.015) (48.8054, 7.7697, 1502.0685) (47.5037, 15.9466, 1503.1219) (44.1062, 23.781, 1504.1752) (39.0264, 30.3195, 1505.2285) (33.9478, 36.8566, 1506.2816) (27.1983, 42.0846, 1507.3347) (19.5991, 45.3675, 1508.3877) (11.7904, 48.7409, 1509.4699) (3.1011, 50.0507, 1510.552) (-5.355, 49.129, 1511.6341) (-13.6173, 48.2284, 1512.6914) (-21.6389, 45.2014, 1513.7487) (-28.4364, 40.4191, 1514.806) (-35.2289, 35.6404, 1515.8625) (-40.7846, 29.1192, 1516.919) (-44.4235, 21.6538, 1517.9756) (-48.06, 14.1935, 1519.0314) (-49.7745, 5.8063, 1520.0872) (-49.3576, -2.4825, 1521.1429) (-48.941, -10.766, 1522.1981) (-46.3965, -18.9338, 1523.2532) (-42.035, -25.9883, 1524.3083) (-37.6761, -33.0388, 1525.3628) (-31.5114, -38.9625, 1526.4173) (-24.2929, -43.0371, 1527.4718) (-17.0783, -47.1095, 1528.5257) (-8.8262, -49.3262, 1529.5796) (-0.5421, -49.417, 1530.6335) (7.738, -49.5079, 1531.6869) (16.0326, -47.4748, 1532.7404) (23.3322, -43.5654, 1533.7938) (30.9937, -39.4621, 1534.8994) (37.5387, -33.2975, 1536.005) (42.0926, -25.895, 1537.1107) (46.4452, -18.8198, 1538.1674) (48.9724, -10.6321, 1539.2242) (49.3648, -2.3346, 1540.2809) (49.7567, 5.9516, 1541.3362) (48.0188, 14.3298, 1542.3915) (44.3635, 21.7765, 1543.4468) (40.7124, 29.2145, 1544.5009) (35.1561, 35.7077, 1545.555) (28.3718, 40.4646, 1546.6091) (21.5939, 45.2169, 1547.6621) (13.6046, 48.2263, 1548.7152) (5.3758, 49.1267, 1549.7683) (-2.874, 50.0295, 1550.824) (-11.3473, 48.8104, 1551.8798) (-19.008, 45.6183, 1552.9356) (-26.6514, 42.4335, 1553.989) (-33.4699, 37.2916, 1555.0423) (-38.6336, 30.8185, 1556.0957) (-43.8008, 24.341, 1557.1498) (-47.3, 16.5441, 1558.2039) (-48.7047, 8.378, 1559.258) (-49.1804, 5.6124, 1559.615) (-49.42, 2.8062, 1559.972) (-49.42, 0, 1560.329) knots 0.40415607 0.40415607 0.40415607 0.40415607 0.50453409 0.50453409 0.50453409 1.00905606 1.00905606 1.00905606 1.51356593 1.51356593 1.51356593 2.01806374 2.01806374 2.01806374 2.5225495 2.5225495 2.5225495 3.02702325 3.02702325 3.02702325 3.53148501 3.53148501 3.53148501 4.0359348 4.0359348 4.0359348 4.54037265 4.54037265 4.54037265 5.04479858 5.04479858 5.04479858 5.54921263 5.54921263 5.54921263 6.05361481 6.05361481 6.05361481 6.55800516 6.55800516 6.55800516 7.06238369 7.06238369 7.06238369 7.56675043 7.56675043 7.56675043 8.07110541 8.07110541 8.07110541 8.57544866 8.57544866 8.57544866 9.0797802 9.0797802 9.0797802 9.58410005 9.58410005 9.58410005 10.08840824 10.08840824 10.08840824 10.5927048 10.5927048 10.5927048 11.09698975 11.09698975 11.09698975 11.60126311 11.60126311 11.60126311 12.10552492 12.10552492 12.10552492 12.60977519 12.60977519 12.60977519 13.11401396 13.11401396 13.11401396 13.61824125 13.61824125 13.61824125 14.12245708 14.12245708 14.12245708 14.62666148 14.62666148 14.62666148 15.13085447 15.13085447 15.13085447 15.63503608 15.63503608 15.63503608 16.13920634 16.13920634 16.13920634 16.64336527 16.64336527 16.64336527 17.1475129 17.1475129 17.1475129 17.65164925 17.65164925 17.65164925 18.15577434 18.15577434 18.15577434 18.65988821 18.65988821 18.65988821 19.16399088 19.16399088 19.16399088 19.66808237 19.66808237 19.66808237 20.1721627 20.1721627 20.1721627 20.67623191 20.67623191 20.67623191 21.18029002 21.18029002 21.18029002 21.68433706 21.68433706 21.68433706 22.18837304 22.18837304 22.18837304 22.692398 22.692398 22.692398 23.19641196 23.19641196 23.19641196 23.70041495 23.70041495 23.70041495 24.20440698 24.20440698 24.20440698 24.70838809 24.70838809 24.70838809 25.21235831 25.21235831 25.21235831 25.71631765 25.71631765 25.71631765 26.22026614 26.22026614 26.22026614 26.72420382 26.72420382 26.72420382 27.22813069 27.22813069 27.22813069 27.73204679 27.73204679 27.73204679 28.23595215 28.23595215 28.23595215 28.73984678 28.73984678 28.73984678 29.24373072 29.24373072 29.24373072 29.74760399 29.74760399 29.74760399 30.25146661 30.25146661 30.25146661 30.75531861 30.75531861 30.75531861 31.25916001 31.25916001 31.25916001 31.76299085 31.76299085 31.76299085 32.26681114 32.26681114 32.26681114 32.77062091 32.77062091 32.77062091 33.27442019 33.27442019 33.27442019 33.778209 33.778209 33.778209 34.28198736 34.28198736 34.28198736 34.78575531 34.78575531 34.78575531 35.28951286 35.28951286 35.28951286 35.79326004 35.79326004 35.79326004 36.29699688 36.29699688 36.29699688 36.8007234 36.8007234 36.8007234 37.30443963 37.30443963 37.30443963 37.80814559 37.80814559 37.80814559 38.31184131 38.31184131 38.31184131 38.81552681 38.81552681 38.81552681 39.31920212 39.31920212 39.31920212 39.82286726 39.82286726 39.82286726 40.32652226 40.32652226 40.32652226 40.83016714 40.83016714 40.83016714 41.33380193 41.33380193 41.33380193 41.83742666 41.83742666 41.83742666 42.34104134 42.34104134 42.34104134 42.84464601 42.84464601 42.84464601 43.34824068 43.34824068 43.34824068 43.85182539 43.85182539 43.85182539 44.35540016 44.35540016 44.35540016 44.85896501 44.85896501 44.85896501 45.36251997 45.36251997 45.36251997 45.86606506 45.86606506 45.86606506 46.36960032 46.36960032 46.36960032 46.87312575 46.87312575 46.87312575 47.3766414 47.3766414 47.3766414 47.88014728 47.88014728 47.88014728 48.38364342 48.38364342 48.38364342 48.88712985 48.88712985 48.88712985 49.39060658 49.39060658 49.39060658 49.89407365 49.89407365 49.89407365 50.39753108 50.39753108 50.39753108 50.90097889 50.90097889 50.90097889 51.40441712 51.40441712 51.40441712 51.90784577 51.90784577 51.90784577 52.41126489 52.41126489 52.41126489 52.91467449 52.91467449 52.91467449 53.4180746 53.4180746 53.4180746 53.92146525 53.92146525 53.92146525 54.42484646 54.42484646 54.42484646 54.92821825 54.92821825 54.92821825 55.43158064 55.43158064 55.43158064 55.93493368 55.93493368 55.93493368 56.43827737 56.43827737 56.43827737 56.94161175 56.94161175 56.94161175 57.44493684 57.44493684 57.44493684 57.94825266 57.94825266 57.94825266 58.45155924 58.45155924 58.45155924 58.95485661 58.95485661 58.95485661 59.45814478 59.45814478 59.45814478 59.96142379 59.96142379 59.96142379 60.46469366 60.46469366 60.46469366 60.96795441 60.96795441 60.96795441 61.47120607 61.47120607 61.47120607 61.97444867 61.97444867 61.97444867 62.47768222 62.47768222 62.47768222 62.98090676 62.98090676 62.98090676 63.4841223 63.4841223 63.4841223 63.98732888 63.98732888 63.98732888 64.49052652 64.49052652 64.49052652 64.99371524 64.99371524 64.99371524 65.49689507 65.49689507 65.49689507 66.00006604 66.00006604 66.00006604 66.50322816 66.50322816 66.50322816 67.00638146 67.00638146 67.00638146 67.50952597 67.50952597 67.50952597 68.01266171 68.01266171 68.01266171 68.51578872 68.51578872 68.51578872 69.018907 69.018907 69.018907 69.52201659 69.52201659 69.52201659 70.02511751 70.02511751 70.02511751 70.52820979 70.52820979 70.52820979 71.03129345 71.03129345 71.03129345 71.53436852 71.53436852 71.53436852 72.03743502 72.03743502 72.03743502 72.54049297 72.54049297 72.54049297 73.04354241 73.04354241 73.04354241 73.54658335 73.54658335 73.54658335 74.04961582 74.04961582 74.04961582 74.55263985 74.55263985 74.55263985 75.05565546 75.05565546 75.05565546 75.55866267 75.55866267 75.55866267 76.06166152 76.06166152 76.06166152 76.56465201 76.56465201 76.56465201 77.06763419 77.06763419 77.06763419 77.57060807 77.57060807 77.57060807 78.07357368 78.07357368 78.07357368 78.57653104 78.57653104 78.57653104 79.07948019 79.07948019 79.07948019 79.58242113 79.58242113 79.58242113 80.0853539 80.0853539 80.0853539 80.58827853 80.58827853 80.58827853 81.09119503 81.09119503 81.09119503 81.59410344 81.59410344 81.59410344 82.09700377 82.09700377 82.09700377 82.59989606 82.59989606 82.59989606 83.10278032 83.10278032 83.10278032 83.60565658 83.60565658 83.60565658 84.10852487 84.10852487 84.10852487 84.61138521 84.61138521 84.61138521 85.11423762 85.11423762 85.11423762 85.61708214 85.61708214 85.61708214 86.11991877 86.11991877 86.11991877 86.62274756 86.62274756 86.62274756 87.12556853 87.12556853 87.12556853 87.62838169 87.62838169 87.62838169 88.13118707 88.13118707 88.13118707 88.63398471 88.63398471 88.63398471 89.13677461 89.13677461 89.13677461 89.63955682 89.63955682 89.63955682 90.14233134 90.14233134 90.14233134 90.64509822 90.64509822 90.64509822 91.14785746 91.14785746 91.14785746 91.65060911 91.65060911 91.65060911 92.15335317 92.15335317 92.15335317 92.65608968 92.65608968 92.65608968 93.15881866 93.15881866 93.15881866 93.66154013 93.66154013 93.66154013 94.16425412 94.16425412 94.16425412 94.66696066 94.66696066 94.66696066 95.16965977 95.16965977 95.16965977 95.67235147 95.67235147 95.67235147 96.17503579 96.17503579 96.17503579 96.67771275 96.67771275 96.67771275 97.18038238 97.18038238 97.18038238 97.6830447 97.6830447 97.6830447 98.18569974 98.18569974 98.18569974 98.68834752 98.68834752 98.68834752 99.19098806 99.19098806 99.19098806 99.6936214 99.6936214 99.6936214 100.19624755 100.19624755 100.19624755 100.69886654 100.69886654 100.69886654 101.20147839 101.20147839 101.20147839 101.70408314 101.70408314 101.70408314 102.20668079 102.20668079 102.20668079 102.70927139 102.70927139 102.70927139 103.21185495 103.21185495 103.21185495 103.71443149 103.71443149 103.71443149 104.21700105 104.21700105 104.21700105 104.71956364 104.71956364 104.71956364 105.2221193 105.2221193 105.2221193 105.72466804 105.72466804 105.72466804 106.22720989 106.22720989 106.22720989 106.72974487 106.72974487 106.72974487 107.23227302 107.23227302 107.23227302 107.73479435 107.73479435 107.73479435 108.23730888 108.23730888 108.23730888 108.73981665 108.73981665 108.73981665 109.24231768 109.24231768 109.24231768 109.74481199 109.74481199 109.74481199 110.2472996 110.2472996 110.2472996 110.74978055 110.74978055 110.74978055 111.25225485 111.25225485 111.25225485 111.75472253 111.75472253 111.75472253 112.25718362 112.25718362 112.25718362 112.75963813 112.75963813 112.75963813 113.2620861 113.2620861 113.2620861 113.78913194 113.78913194 113.78913194 114.314119 114.314119 114.314119 114.83705533 114.83705533 114.83705533 115.35794894 115.35794894 115.35794894 115.87680781 115.87680781 115.87680781 116.39363989 116.39363989 116.39363989 116.90845309 116.90845309 116.90845309 117.4212553 117.4212553 117.4212553 117.93205438 117.93205438 117.93205438 118.44085815 118.44085815 118.44085815 118.94767441 118.94767441 118.94767441 119.45251091 119.45251091 119.45251091 119.95727245 119.95727245 119.95727245 120.46200882 120.46200882 120.46200882 120.96672014 120.96672014 120.96672014 121.47140652 121.47140652 121.47140652 121.97606804 121.97606804 121.97606804 122.48070482 122.48070482 122.48070482 122.98531696 122.98531696 122.98531696 123.48990455 123.48990455 123.48990455 123.99446771 123.99446771 123.99446771 124.49900654 124.49900654 124.49900654 125.00352113 125.00352113 125.00352113 125.50801159 125.50801159 125.50801159 126.01247802 126.01247802 126.01247802 126.51692052 126.51692052 126.51692052 127.0213392 127.0213392 127.0213392 127.52573416 127.52573416 127.52573416 128.0301055 128.0301055 128.0301055 128.53445332 128.53445332 128.53445332 129.03877773 129.03877773 129.03877773 129.54307882 129.54307882 129.54307882 130.0473567 130.0473567 130.0473567 130.55161147 130.55161147 130.55161147 131.05584323 131.05584323 131.05584323 131.56005208 131.56005208 131.56005208 132.06423813 132.06423813 132.06423813 132.56840147 132.56840147 132.56840147 133.07254222 133.07254222 133.07254222 133.57666046 133.57666046 133.57666046 134.0807563 134.0807563 134.0807563 134.58482984 134.58482984 134.58482984 135.08888119 135.08888119 135.08888119 135.59291044 135.59291044 135.59291044 136.0969177 136.0969177 136.0969177 136.60090307 136.60090307 136.60090307 137.10486664 137.10486664 137.10486664 137.60880853 137.60880853 137.60880853 138.11272883 138.11272883 138.11272883 138.61662763 138.61662763 138.61662763 139.12050505 139.12050505 139.12050505 139.62436119 139.62436119 139.62436119 140.12819614 140.12819614 140.12819614 140.63201001 140.63201001 140.63201001 141.13580289 141.13580289 141.13580289 141.63957489 141.63957489 141.63957489 142.1433261 142.1433261 142.1433261 142.64705664 142.64705664 142.64705664 143.1507666 143.1507666 143.1507666 143.65445607 143.65445607 143.65445607 144.15812517 144.15812517 144.15812517 144.66177399 144.66177399 144.66177399 145.16540263 145.16540263 145.16540263 145.66901119 145.66901119 145.66901119 146.17259978 146.17259978 146.17259978 146.67616849 146.67616849 146.67616849 147.17971742 147.17971742 147.17971742 147.68324667 147.68324667 147.68324667 148.18675635 148.18675635 148.18675635 148.69024656 148.69024656 148.69024656 149.19371738 149.19371738 149.19371738 149.69716894 149.69716894 149.69716894 150.20060131 150.20060131 150.20060131 150.70401461 150.70401461 150.70401461 151.20740894 151.20740894 151.20740894 151.71078439 151.71078439 151.71078439 152.21414106 152.21414106 152.21414106 152.71747906 152.71747906 152.71747906 153.22079849 153.22079849 153.22079849 153.72409943 153.72409943 153.72409943 154.22738201 154.22738201 154.22738201 154.7306463 154.7306463 154.7306463 155.23389242 155.23389242 155.23389242 155.73712046 155.73712046 155.73712046 156.24033052 156.24033052 156.24033052 156.74352271 156.74352271 156.74352271 157.24669712 157.24669712 157.24669712 157.74985385 157.74985385 157.74985385 158.252993 158.252993 158.252993 158.75611467 158.75611467 158.75611467 159.25921896 159.25921896 159.25921896 159.76230596 159.76230596 159.76230596 160.26537579 160.26537579 160.26537579 160.76842854 160.76842854 160.76842854 161.2714643 161.2714643 161.2714643 161.77448318 161.77448318 161.77448318 162.27748527 162.27748527 162.27748527 162.78047068 162.78047068 162.78047068 163.2834395 163.2834395 163.2834395 163.78639183 163.78639183 163.78639183 164.28932778 164.28932778 164.28932778 164.79224744 164.79224744 164.79224744 165.2951509 165.2951509 165.2951509 165.79803828 165.79803828 165.79803828 166.30090966 166.30090966 166.30090966 166.80376515 166.80376515 166.80376515 167.30660485 167.30660485 167.30660485 167.80942885 167.80942885 167.80942885 168.31223725 168.31223725 168.31223725 168.81503016 168.81503016 168.81503016 169.31780766 169.31780766 169.31780766 169.82056987 169.82056987 169.82056987 170.32331687 170.32331687 170.32331687 170.82604877 170.82604877 170.82604877 171.32876567 171.32876567 171.32876567 171.83146766 171.83146766 171.83146766 172.33415484 172.33415484 172.33415484 172.83682732 172.83682732 172.83682732 173.33948518 173.33948518 173.33948518 173.84212853 173.84212853 173.84212853 174.34475747 174.34475747 174.34475747 174.84737209 174.84737209 174.84737209 175.3499725 175.3499725 175.3499725 175.85255879 175.85255879 175.85255879 176.35513105 176.35513105 176.35513105 176.8576894 176.8576894 176.8576894 177.36023392 177.36023392 177.36023392 177.86276472 177.86276472 177.86276472 178.36528189 178.36528189 178.36528189 178.86778553 178.86778553 178.86778553 179.37027574 179.37027574 179.37027574 179.87275262 179.87275262 179.87275262 180.37521626 180.37521626 180.37521626 180.87766677 180.87766677 180.87766677 181.40351171 181.40351171 181.40351171 181.9252485 181.9252485 181.9252485 182.44290921 182.44290921 182.44290921 182.9565257 182.9565257 182.9565257 183.46612955 183.46612955 183.46612955 183.97175213 183.97175213 183.97175213 184.47649844 184.47649844 184.47649844 184.98119467 184.98119467 184.98119467 185.48584122 185.48584122 185.48584122 185.9904385 185.9904385 185.9904385 186.49498693 186.49498693 186.49498693 186.99948691 186.99948691 186.99948691 187.50393886 187.50393886 187.50393886 188.00834318 188.00834318 188.00834318 188.51270028 188.51270028 188.51270028 189.01701057 189.01701057 189.01701057 189.52127445 189.52127445 189.52127445 190.02549234 190.02549234 190.02549234 190.52966463 190.52966463 190.52966463 191.03379175 191.03379175 191.03379175 191.53787408 191.53787408 191.53787408 192.04191204 192.04191204 192.04191204 192.54590604 192.54590604 192.54590604 193.04985647 193.04985647 193.04985647 193.55376374 193.55376374 193.55376374 194.05762827 194.05762827 194.05762827 194.56145044 194.56145044 194.56145044 195.06523066 195.06523066 195.06523066 195.56896934 195.56896934 195.56896934 196.07266688 196.07266688 196.07266688 196.57632369 196.57632369 196.57632369 197.07994016 197.07994016 197.07994016 197.58351669 197.58351669 197.58351669 198.08705369 198.08705369 198.08705369 198.59055156 198.59055156 198.59055156 199.09401069 199.09401069 199.09401069 199.5974315 199.5974315 199.5974315 200.10081438 200.10081438 200.10081438 200.60415972 200.60415972 200.60415972 201.10746794 201.10746794 201.10746794 201.61073942 201.61073942 201.61073942 202.11397457 202.11397457 202.11397457 202.61717379 202.61717379 202.61717379 203.12033747 203.12033747 203.12033747 203.62346601 203.62346601 203.62346601 204.12655981 204.12655981 204.12655981 204.62961927 204.62961927 204.62961927 205.13264478 205.13264478 205.13264478 205.63563675 205.63563675 205.63563675 206.13859556 206.13859556 206.13859556 206.64152162 206.64152162 206.64152162 207.14441531 207.14441531 207.14441531 207.64727705 207.64727705 207.64727705 208.15010721 208.15010721 208.15010721 208.6529062 208.6529062 208.6529062 209.15567442 209.15567442 209.15567442 209.65841225 209.65841225 209.65841225 210.16112009 210.16112009 210.16112009 210.66379834 210.66379834 210.66379834 211.16644738 211.16644738 211.16644738 211.66906763 211.66906763 211.66906763 212.17165945 212.17165945 212.17165945 212.67422326 212.67422326 212.67422326 213.17675945 213.17675945 213.17675945 213.67926839 213.67926839 213.67926839 214.1817505 214.1817505 214.1817505 214.68420616 214.68420616 214.68420616 215.20766887 215.20766887 215.20766887 215.72295248 215.72295248 215.72295248 216.23018478 216.23018478 216.23018478 216.73490099 216.73490099 216.73490099 217.23951793 217.23951793 217.23951793 217.74403724 217.74403724 217.74403724 218.24846056 218.24846056 218.24846056 218.75278951 218.75278951 218.75278951 219.25702573 219.25702573 219.25702573 219.76117084 219.76117084 219.76117084 220.26522648 220.26522648 220.26522648 220.76919426 220.76919426 220.76919426 221.27307581 221.27307581 221.27307581 221.77687273 221.77687273 221.77687273 222.28058664 222.28058664 222.28058664 222.78421915 222.78421915 222.78421915 223.28777188 223.28777188 223.28777188 223.79124642 223.79124642 223.79124642 224.29464437 224.29464437 224.29464437 224.79796734 224.79796734 224.79796734 225.30121693 225.30121693 225.30121693 225.80439472 225.80439472 225.80439472 226.30750232 226.30750232 226.30750232 226.81054131 226.81054131 226.81054131 227.31351329 227.31351329 227.31351329 227.81641982 227.81641982 227.81641982 228.31926251 228.31926251 228.31926251 228.82204294 228.82204294 228.82204294 229.32476267 229.32476267 229.32476267 229.82742329 229.82742329 229.82742329 230.33002638 230.33002638 230.33002638 230.83257351 230.83257351 230.83257351 231.33506625 231.33506625 231.33506625 231.8616523 231.8616523 231.8616523 232.37178253 232.37178253 232.37178253 232.87643413 232.87643413 232.87643413 233.38089093 233.38089093 233.38089093 233.88515948 233.88515948 233.88515948 234.38924629 234.38924629 234.38924629 234.89315786 234.89315786 234.89315786 235.39690065 235.39690065 235.39690065 235.90048112 235.90048112 235.90048112 236.40390568 236.40390568 236.40390568 236.90718074 236.90718074 236.90718074 237.41031269 237.41031269 237.41031269 237.9133079 237.9133079 237.9133079 238.4161727 238.4161727 238.4161727 238.91891345 238.91891345 238.91891345 239.42153644 239.42153644 239.42153644 239.92404797 239.92404797 239.92404797 240.4404087 240.4404087 240.4404087 240.9449348 240.9449348 240.9449348 241.44908614 241.44908614 241.44908614 241.95288875 241.95288875 241.95288875 242.45636847 242.45636847 242.45636847 242.95955095 242.95955095 242.95955095 243.4624617 243.4624617 243.4624617 243.96512609 243.96512609 243.96512609 244.49271278 244.49271278 244.49271278 244.99696942 244.99696942 244.99696942 245.50053931 245.50053931 245.50053931 246.0035254 246.0035254 246.0035254 246.50602939 246.50602939 246.50602939 247.00982031 247.00982031 247.00982031 247.51247571 247.51247571 247.51247571 248.01547038 248.01547038 248.01547038 248.18581963 248.18581963 248.18581963 248.18581963